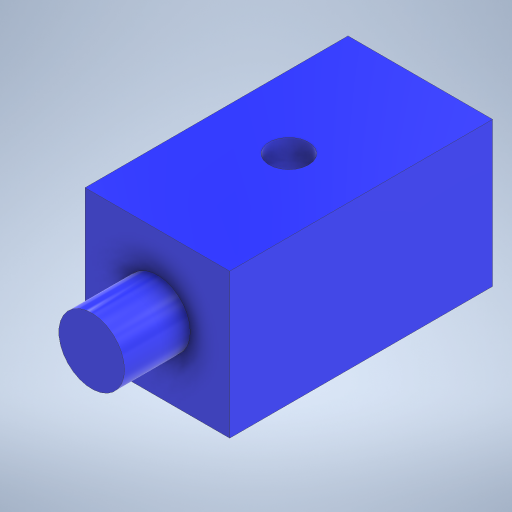
# Autodesk Inventor part: Aluminium-Connector_Lengan pendek
Saved by Autodesk Inventor 2024 (Build 280153000, 153)
## iProperties
Created: 2023-09-10
Part Number: Aluminium-Connector_Lengan pendek
Material: Generic
Document SubType Name: Modeling
Designer: AlfaNooraFithria
Density: 1 g/cm^3
Appearance: Default
Author: AlfaNooraFithria
Autodesk Inventor part; units mm, degrees
ref_plane "YZ Plane" through (0, 0, 0) normal (1, 0, 0) x (0, 1, 0)
ref_plane "XZ Plane" through (0, 0, 0) normal (0, 1, 0) x (-1, 0, 0)
ref_plane "XY Plane" through (0, 0, 0) normal (0, 0, 1) x (1, 0, 0)
sketch "Sketch1" plane through (0, 0, 0) normal (0, 0, 1) x (1, 0, 0)
  line L0 (0, 0) -> (11, 0)
  line L1 (11, 0) -> (11, 11)
  line L2 (11, 11) -> (0, 11)
  line L3 (0, 11) -> (0, 0)
  dimension "d0" = 11
  dimension "d1" = 11
  constraints: 8 end point, 2 parallel, 1 horizontal, 1 perpendicular
  measures "d0" distance of L2.end L1.end
  measures "d1" distance of L1.end L0.end
extrude "Extrusion1" add sketch "Sketch1" against normal blind 20
sketch "Sketch2" plane through (0, 0, 0) normal (0, 0, 1) x (1, 0, 0)
  line L0 (0, 0) -> (0, 11) projected
  line L1 (11, 11) -> (11, 0) projected
  line L2 (0, 11) -> (11, 0)
  line L3 (11, 0) -> (11, 11)
  line L4 (11, 11) -> (0, 0)
  circle A0 centre (5.5, 5.5) radius 2.5
  dimension "d4" = 5
  constraints: 6 end point, 1 centre point, 1 collinear, 1 midpoint, 1 perpendicular
  measures "d4" diameter of A0
extrude "Extrusion2" add sketch "Sketch2" along normal blind 5 contours A0 L2 L4 | L4 L2 A0 | A0 L4 L2 | L4 A0 L2
sketch "Sketch3" plane through (0, 11, 0) normal (0, 1, 0) x (1, 0, 0)
  line L0 (0, 0) -> (0, 20) projected
  line L1 (0, 10) -> (11, 10)
  line L2 (11, 0) -> (11, 20) projected
  line L3 (0, 0) -> (11, 0) projected
  line L4 (5.5, 0) -> (5.5, 20)
  circle A0 centre (5.5, 10) radius 1.5
  dimension "d7" = 3
  constraints: 4 end point, 4 midpoint, 1 centre point, 1 vertical
  measures "d7" diameter of A0
extrude "Extrusion3" cut sketch "Sketch3" against normal through all contours A0 L4 L1 | L1 L4 A0 | L4 L1 A0 | L4 A0 L1
body "Solid1"
